Biokuebel_Klammer_v2 (Autodesk Fusion 360 design; units mm, degrees)
Autodesk Fusion 360 part; units mm, degrees
note: some values were not read from the file. Set by a fixed rule: which face or edge a step refers to.
sketch "Sketch1" plane through (0, 0, 0) normal (0, 1, 0) x (1, 0, 0)
  circle A0 centre (5, -5.25) radius 7.25
  line L0 (10, 0) -> (10, -11.75)
  line L1 (10, -11.75) -> (7.8, -11.75)
  line L2 (7.8, -11.75) -> (7.8, -7.75)
  line L3 (7.8, -7.75) -> (6, -7.75)
  line L4 (6, -7.75) -> (6, -13.75)
  line L5 (6, -13.75) -> (12, -13.75)
  line L6 (12, -13.75) -> (12, 1)
  line L7 (0, 0) -> (-1, 0)
  line L8 (-1, 0) -> (-1, 1)
  circle A1 centre (5.5, -4.2583) radius 8.3606
  dimension "d5" = 2.2
  dimension "d6" = 11.75
  dimension "d8" = 4
  dimension "d9" = 2
  constraint coincident L7.start A0
  constraint coincident A0 L0.start
  constraint vertical L0
  constraint perpendicular L0 L1
  constraint perpendicular L1 L2
  constraint perpendicular L2 L3
  constraint perpendicular L3 L4
  constraint perpendicular L4 L5
  constraint perpendicular L3 L6
  constraint coincident L7.start origin
  constraint horizontal L7
  constraint perpendicular L7 L8
  constraint coincident L8.end A1
  constraint coincident L6.end A1
  constraint tangent A0 A1
  measures "d5" distance of L0.end L1.end
  measures "d6" distance of L0.start L0.end
  measures "d8" distance of L1 L3
  measures "d9" distance of L1 L5
ref_plane "WorkPlane1" through (-100, 0, 0) normal (1, 0, 0) x (0, 1, 0)
revolve "Revolve1" add sketch "Sketch1" angle 25 about axis through (-100, 0, -5.1704) along (0, 0, 1) contours A0 L6 L7 L8 A1 | A0 L0 L6 | A0 L0 L6 A1 | A0 L1 L4 A1 | A0 L1 L2 L3 L4 | L0 L1 L4 L5 L6 A1
fillet "Fillet2" radius 0.5 33 edges at (9.3452, 24.2412, -1) (9, 0, 13.75) (7.8, 0, 9.75) (3.4874, 22.9426, 7.75) (-1.2125, 46.0654, 13.75) (-3.1157, 45.1779, 7.75) (-3.9314, 44.7975, 10.75) (-1, 0, -0.5) (-10.2755, 41.8392, -0.5) (7.3926, 23.8084, 11.75) (7.3926, 23.8084, 0) (-2.3704, 21.644, 0) (-9.8224, 42.0505, 0) (-0.3061, 46.488, 5.875) (8.9, 0, 11.75) (-0.5, 0, 0) (-3.3467, 21.4275, 0) (12, 0, 6.375) (-4.8377, 44.3749, -2) (5.5, 0, -4.1023) (10, 0, 5.875) (-3.3467, 21.4275, -1) (5, 0, -2) (9.3452, 24.2412, 13.75) (-4.3845, 44.5862, -4.1023) (-1.3031, 46.0231, 11.75) (5.2447, 23.3322, 11.75) (6.9, 0, 7.75) (6, 0, 10.75) (3.4874, 22.9426, 13.75) (1.5065, 47.3332, 6.375) (-2.3, 45.5582, 9.75) (5.2447, 23.3322, 7.75) 13 faces at (11.4739, 10.8428, 12.3389) (5.3593, 37.1948, -1.315) (-2.4341, 19.1739, 0) (9.8708, 5.3309, 7) (6.8206, 5.2079, 7.75) (0.2981, 46.7698, 5.8792) (5.7793, 20.7744, 9.0833) (-1.465, 9.5843, -0.3333) (1.6233, 41.4176, 13.75) (7.4252, 21.1064, 11.75) (9.2371, 10.6252, -0.2249) (10.6667, 0, 5.8792) (2.9009, 25.4442, 9.3102)
extrude "Extrude1" [suppressed]
fillet "Fillet1" [suppressed]
